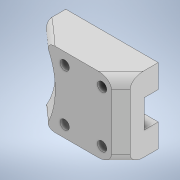
# Autodesk Inventor part: armtip_2_mod
Saved by Autodesk Inventor 2020 (Build 240168000, 168)
## iProperties
Created: 2019-10-15
Part Number: armtip_2_mod
Material: Generic
Document SubType Name: Modeling
Designer: psrob
Density: 1 g/cm^3
Appearance: Default
Author: psrob
Autodesk Inventor part; units mm, degrees
ref_plane "YZ Plane" through (0, 0, 0) normal (1, 0, 0) x (0, 1, 0)
ref_plane "XZ Plane" through (0, 0, 0) normal (0, 1, 0) x (-1, 0, 0)
ref_plane "XY Plane" through (0, 0, 0) normal (0, 0, 1) x (1, 0, 0)
sketch "Sketch1" plane through (0, 0, 0) normal (0, 0, 1) x (1, 0, 0)
  circle A0 centre (-0.7749, 5.5) radius 1 projected
  circle A1 centre (7.2251, 5.5) radius 1 projected
  circle A2 centre (-0.7749, -5.5) radius 1 projected
  circle A3 centre (7.2251, -5.5) radius 1 projected
  line L0 (11.2251, -3) -> (-3.7749, -3) projected
  line L1 (-3.7749, -3) -> (-3.7749, 3) projected
  line L2 (-3.7749, 3) -> (11.2251, 3) projected
  line L3 (11.2251, 3) -> (11.2251, 8) projected
  line L4 (11.2251, 8) -> (-8.528, 8) projected
  arc A4 (-8.528, -8) -> (-8.528, 8) centre (-18.7749, 0) ccw projected
  line L5 (-8.528, -8) -> (11.2251, -8) projected
  line L6 (11.2251, -8) -> (11.2251, -3) projected
  point P0 (0, 0)
extrude "Extrusion1" add sketch "Sketch1" along normal blind 3
sketch "Sketch2" plane through (0, 0, 3) normal (0, 0, 1) x (1, 0, 0)
  line L0 (11.2251, -8) -> (11.2251, -3) projected
  line L1 (11.2251, -3) -> (-3.7749, -3) projected
  line L2 (-3.7749, -3) -> (-3.7749, 3) projected
  line L3 (-3.7749, 3) -> (11.2251, 3) projected
  line L4 (11.2251, 3) -> (11.2251, 8) projected
  line L5 (11.2251, 8) -> (-8.528, 8) projected
  arc A0 (-8.528, -8) -> (-8.528, 8) centre (-18.7749, 0) ccw projected
  line L6 (-8.528, -8) -> (11.2251, -8) projected
  circle A1 centre (-0.7749, 5.5) radius 1 projected
  circle A2 centre (7.2251, 5.5) radius 1 projected
  circle A3 centre (-0.7749, -5.5) radius 1 projected
  circle A4 centre (7.2251, -5.5) radius 1 projected
  line L7 (11.2251, -8) -> (11.2251, -3) projected
  line L8 (11.2251, 3) -> (11.2251, 8) projected
  line L9 (11.2251, -8) -> (11.2251, 8)
  point P0 (0, 0)
  constraints: 2 end point, 1 collinear
extrude "Extrusion2" add sketch "Sketch2" along normal blind 5
chamfer "Chamfer1" distance 3 angle 45 1 edges at (-5.7749, 0, 8)
fillet "Fillet1" radius 1 2 edges at (-6.817, -8, 6.3872) (-6.817, 8, 6.3872)
chamfer "Chamfer2" distance 2 angle 45 1 edges at (11.2251, 0, 8)
fillet "Fillet2" radius 2 2 edges at (10.2251, -8, 7) (10.2251, 8, 7)
body "Solid1"
